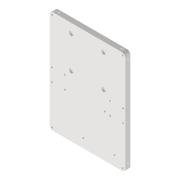
# Autodesk Inventor part: Omniscope_USBC_Base
Saved by Autodesk Inventor 2022 (Build 260153000, 153)
## iProperties
Created: 2023-05-17
Part Number: Omniscope_USBC_Base
Material: Generisch
Document SubType Name: Modeling
Designer: diederichbenedict
Density: 1 g/cm^3
Appearance: Vorgabe
Author: diederichbenedict
Autodesk Inventor part; units mm, degrees
ref_plane "YZ Plane" through (0, 0, 0) normal (1, 0, 0) x (0, 1, 0)
ref_plane "XZ Plane" through (0, 0, 0) normal (0, 1, 0) x (-1, 0, 0)
ref_plane "XY Plane" through (0, 0, 0) normal (0, 0, 1) x (1, 0, 0)
ref_plane "Arbeitsebene1" through (0, 0, 0) normal (0, 0, 1) x (1, 0, 0)
sketch "Skizze1" plane through (0, 0, 0) normal (0, 0, 1) x (1, 0, 0)
  point P0 (0, 0)
ref_plane "Arbeitsebene2" through (0, 0, 0) normal (0, 0, 1) x (1, 0, 0)
sketch "Skizze2" plane through (0, 0, 0) normal (0, 0, 1) x (1, 0, 0)
  line L0 (58.4152, -114.421) -> (58.4152, 34.421) projected
  arc A0 (58.4152, 34.421) -> (53.4152, 39.421) centre (53.4152, 34.421) ccw projected
  line L1 (53.4152, 39.421) -> (-53.4152, 39.421) projected
  arc A1 (-53.4152, 39.421) -> (-58.4152, 34.421) centre (-53.4152, 34.421) ccw projected
  line L2 (-58.4152, 34.421) -> (-58.4152, -114.421) projected
  arc A2 (-58.4152, -114.421) -> (-53.4152, -119.421) centre (-53.4152, -114.421) ccw projected
  line L3 (-53.4152, -119.421) -> (53.4152, -119.421) projected
  arc A3 (53.4152, -119.421) -> (58.4152, -114.421) centre (53.4152, -114.421) ccw projected
  circle A4 centre (-25, 25) radius 2.25 projected
  circle A5 centre (25, 25) radius 2.25 projected
  circle A6 centre (-25, -25) radius 2.25 projected
  circle A7 centre (25, -25) radius 2.25 projected
  circle A8 centre (-54.4152, 35.421) radius 1.4 projected
  circle A9 centre (54.4152, -115.421) radius 1.4 projected
  circle A10 centre (54.4152, 35.421) radius 1.4 projected
  circle A11 centre (-54.4152, -115.421) radius 1.4 projected
  line L4 (41.1596, -107.1216) -> (-37.8004, -107.1216) projected
  line L5 (-37.8004, -107.1216) -> (-37.8004, 14.1284) projected
  line L6 (-37.8004, 14.1284) -> (41.1596, 14.1284) projected
  line L7 (41.1596, 14.1284) -> (41.1596, -107.1216) projected
  point P0 (0, 0)
extrude "Extrusion1" add sketch "Skizze2" along normal blind 8 contours A3 L3 A2 L2 A1 L1 A0 L0 | A4 | A5 | A6 | A7 | A8 | A9 | A10 | A11 | L4 L5 L6 L7
sketch "Skizze4" plane through (0, 0, 8) normal (0, 0, 1) x (1, 0, 0)
  arc A0 (58.4152, 34.421) -> (53.4152, 39.421) centre (53.4152, 34.421) ccw projected
  line L0 (53.4152, 39.421) -> (-53.4152, 39.421) projected
  arc A1 (-53.4152, 39.421) -> (-58.4152, 34.421) centre (-53.4152, 34.421) ccw projected
  line L1 (-58.4152, 34.421) -> (-58.4152, -114.421) projected
  arc A2 (-58.4152, -114.421) -> (-53.4152, -119.421) centre (-53.4152, -114.421) ccw projected
  line L2 (-53.4152, -119.421) -> (53.4152, -119.421) projected
  arc A3 (53.4152, -119.421) -> (58.4152, -114.421) centre (53.4152, -114.421) ccw projected
  line L3 (58.4152, -114.421) -> (58.4152, 34.421) projected
  line L4 (-55, -55) -> (-35, -55)
  line L5 (-35, -55) -> (-35, -35)
  line L6 (-35, -35) -> (-55, -35)
  line L7 (-55, -35) -> (-55, -55)
  line L8 (-55, -55) -> (-35, -35) construction
  line L9 (-35, -55) -> (-55, -35) construction
  line L10 (35, -55) -> (55, -55)
  line L11 (55, -55) -> (55, -35)
  line L12 (55, -35) -> (35, -35)
  line L13 (35, -35) -> (35, -55)
  line L14 (35, -55) -> (55, -35) construction
  line L15 (55, -55) -> (35, -35) construction
  point P0 (0, 0)
  point P1 (-45, -45)
  point P2 (45, -45)
  dimension "d13" = 20
  dimension "d14" = 20
  dimension "d15" = 20
  dimension "d16" = 20
  constraints: 24 end point, 8 coincident, 4 midpoint, 4 parallel, 2 horizontal, 2 perpendicular
  measures "d13" distance of L6.end L5.end
  measures "d14" distance of L5.end L4.end
  measures "d15" distance of L12.end L11.end
  measures "d16" distance of L11.end L10.end
hole "Bohrung1" at (-35, -55, 8) at (-35, -35, 8) at (-55, -35, 8) at (-55, -55, 8) at (35, -55, 8) at (35, -35, 8) at (55, -55, 8) at (55, -35, 8) direction (0, 0, -1) diameter 2.8 end through all
sketch "Skizze5" plane through (0, 0, 8) normal (0, 0, 1) x (1, 0, 0)
  line L0 (-29.2, 30) -> (29.2, 30) projected
  line L1 (-29.2, 30) -> (-30, 29.2) projected
  line L2 (-30, -29.2) -> (-30, 29.2) projected
  line L3 (-30, -29.2) -> (-29.2, -30) projected
  line L4 (-29.2, -30) -> (29.2, -30) projected
  line L5 (29.2, -30) -> (30, -29.2) projected
  line L6 (30, -29.2) -> (30, 29.2) projected
  line L7 (30, 29.2) -> (29.2, 30) projected
  circle A0 centre (-25, -25) radius 2.25 projected
  circle A1 centre (25, -25) radius 2.25 projected
  circle A2 centre (25, 25) radius 2.25 projected
  circle A3 centre (-25, 25) radius 2.25 projected
  point P0 (0, 0)
hole "Bohrung2" at (-25, -25, 8) at (-25, 25, 8) at (25, 25, 8) at (25, -25, 8) direction (0, 0, -1) diameter 2.8 end through all counterbore diameter 6.5 counterbore depth 3
sketch "Skizze6" plane through (-58.4152, -114.421, 0) normal (-1, 0, 0) x (0, 0, 1)
  line L0 (0, 148.842) -> (0, 0) projected
  line L1 (0, 0) -> (8, 0) projected
  line L2 (8, 148.842) -> (8, 0) projected
  line L3 (0, 148.842) -> (8, 148.842) projected
  circle A0 centre (4, 5) radius 1.4
  circle A1 centre (4, 143.842) radius 1.4
  point P0 (0, 114.421)
  dimension "d52" = 2.8
  dimension "d53" = 2.8
  dimension "d54" = 5
  dimension "d55" = 5
  dimension "d68" = 4
  dimension "d69" = 0
  constraints: 2 centre point
  measures "d52" diameter of A0
  measures "d53" diameter of A1
  measures "d54" distance from line of A0.centre L1
  measures "d55" distance from line of L3 A1.centre
  measures "d68" distance from line of A0.centre L0
  measures "d69" horizontal distance of A1.centre A0.centre
extrude "Extrusion3" cut sketch "Skizze6" against normal blind 10 contours A0 | A1
sketch "Skizze7" plane through (-53.4152, 39.421, 0) normal (0, 1, 0) x (1, 0, 0)
  line L0 (106.8304, 0) -> (0, 0) projected
  line L1 (0, 0) -> (0, -8) projected
  line L2 (106.8304, -8) -> (0, -8) projected
  line L3 (106.8304, 0) -> (106.8304, -8) projected
  circle A0 centre (5, -4) radius 1.4
  circle A1 centre (101.8304, -4) radius 1.4
  point P0 (53.4152, 0)
  dimension "d58" = 2.8
  dimension "d59" = 2.8
  dimension "d60" = 5
  dimension "d61" = 5
  dimension "d70" = 4
  dimension "d71" = 4
  constraints: 2 centre point
  measures "d58" diameter of A0
  measures "d59" diameter of A1
  measures "d60" distance from line of A0.centre L1
  measures "d61" distance from line of A1.centre L3
  measures "d70" distance from line of A0.centre L0
  measures "d71" distance from line of A1.centre L0
extrude "Extrusion4" cut sketch "Skizze7" against normal blind 10 contours A0 | A1
sketch "Skizze8" plane through (58.4152, -114.421, 0) normal (1, 0, 0) x (0, 0, -1)
  circle A0 centre (-4, 143.842) radius 1.4 projected
  circle A1 centre (-4, 5) radius 1.4 projected
  line L0 (0, 148.842) -> (0, 0) projected
  line L1 (0, 0) -> (-8, 0) projected
  line L2 (-8, 148.842) -> (-8, 0) projected
  line L3 (0, 148.842) -> (-8, 148.842) projected
  point P0 (0, 114.421)
extrude "Extrusion5" cut sketch "Skizze8" against normal blind 10 contours A0 | A1
sketch "Skizze9" plane through (-53.4152, -119.421, 0) normal (0, -1, 0) x (1, 0, 0)
  circle A0 centre (101.8304, 4) radius 1.4 projected
  circle A1 centre (5, 4) radius 1.4 projected
  line L0 (106.8304, 0) -> (0, 0) projected
  line L1 (0, 0) -> (0, 8) projected
  line L2 (106.8304, 8) -> (0, 8) projected
  line L3 (106.8304, 0) -> (106.8304, 8) projected
  point P0 (53.4152, 0)
extrude "Extrusion6" cut sketch "Skizze9" against normal blind 10 contours A0 | A1
sketch "Skizze10" plane through (0, 0, 0) normal (0, 0, -1) x (-1, 0, 0)
  circle A0 centre (-41.8952, -104.1931) radius 1.75 projected
  circle A1 centre (6.3648, -105.4631) radius 1.75 projected
  circle A2 centre (-26.6552, -53.3931) radius 1.75 projected
  point P0 (0, 0)
hole "Bohrung3" at (26.6552, -53.3931, 0) at (41.8952, -104.1931, 0) at (-6.3648, -105.4631, 0) direction (0, 0, 1) diameter 2.8 end through all counterbore diameter 6.5 counterbore depth 4
equation "\"d68\" = 0.5 * a1"
equation "\"d70\" = 0.5 * a1"
equation "\"d71\" = 0.5 * a1"
equation "\"a1\" = 8"
